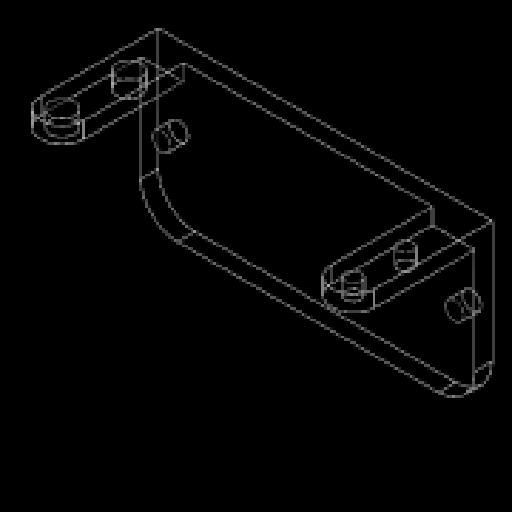
# Autodesk Inventor part: M3RCServoMountBracket
Saved by Autodesk Inventor 2025.2 (Build 292293000, 293)
## iProperties
Created: 2025-12-06
Part Number: M3RCServoMountBracket
Material: Generic
Document SubType Name: Modeling
Designer: valer
Density: 1 g/cm^3
Appearance: Default
Author: valer
Comments: https://www.amazon.com/dp/B0F372CLN4?ref=ppx_yo2ov_dt_b_fed_asin_title
Autodesk Inventor part; units mm, degrees
ref_plane "YZ Plane" through (0, 0, 0) normal (1, 0, 0) x (0, 1, 0)
ref_plane "XZ Plane" through (0, 0, 0) normal (0, 1, 0) x (-1, 0, 0)
ref_plane "XY Plane" through (0, 0, 0) normal (0, 0, 1) x (1, 0, 0)
sketch "Base" plane through (0, 0, 0) normal (0, 0, 1) x (1, 0, 0)
  line L0 (27.5, -13) -> (-27.5, -13)
  line L1 (-27.5, -13) -> (-27.5, 13)
  line L2 (-27.5, 13) -> (27.5, 13)
  line L3 (27.5, 13) -> (27.5, -13)
  line L4 (27.5, -13) -> (-27.5, 13) construction
  line L5 (-27.5, -13) -> (27.5, 13) construction
  line L6 (-27.5, 0) -> (27.5, 0) construction
  circle A0 centre (-24.15, 0) radius 1.5
  line L7 (0, -18.2) -> (0, 18.2) construction
  line L8 (-25.65, -1.5) -> (-22.65, -1.5) construction
  line L9 (-22.65, -1.5) -> (-22.65, 1.5)
  line L10 (-22.65, 1.5) -> (-25.65, 1.5) construction
  line L11 (-25.65, 1.5) -> (-25.65, -1.5) construction
  line L12 (-25.65, -1.5) -> (-22.65, 1.5) construction
  line L13 (-22.65, -1.5) -> (-25.65, 1.5) construction
  circle A1 centre (24.15, 0) radius 1.5
  point P0 (0, 0)
  dimension "d0" = 55
  dimension "d1" = 26
  dimension "d4" = 3
  dimension "d5" = 1.85
  constraints: 26 end point, 6 midpoint, 4 parallel, 2 centre point, 2 perpendicular, 2 tangent, 1 horizontal, 1 point on line, 1 symmetric about line, 1 other
  measures "d0" distance of L0.start L0.end
  measures "d1" distance of L0.end L1.end
  measures "d4" diameter of A0
  measures "d5" distance between parallel lines of L1 L11
extrude "BaseFeature" add sketch "Base" along normal blind 2.88
fillet "BaseFilletsFeature" radius 6 2 edges at (-27.5, -13, 1.44) (27.5, -13, 1.44)
sketch "ServoMount" plane through (0, 0, 2.88) normal (0, 0, 1) x (1, 0, 0)
  line L0 (27.5, 13) -> (-27.5, 13) projected
  line L1 (-27.5, 13) -> (-27.5, -7) projected
  line L2 (27.5, -7) -> (27.5, 13) projected
  line L3 (-27.5, 13) -> (-20.5, 13)
  line L4 (-20.5, 13) -> (-20.5, 10.35)
  line L5 (-20.5, 10.35) -> (-27.5, 10.35)
  line L6 (-27.5, 10.35) -> (-27.5, 13)
  line L7 (0, -18.2) -> (0, 18.2) construction
  line L8 (20.5, 13) -> (20.5, 10.35)
  line L9 (20.5, 10.35) -> (27.5, 10.35)
  point P0 (0, 0)
  point P1 (-24, 13)
  dimension "d7" = 2.65
  dimension "d8" = 7
  constraints: 12 end point, 3 symmetric about line, 2 parallel, 1 horizontal, 1 midpoint, 1 perpendicular
  measures "d7" distance from line of point (-24, 13) L5
  measures "d8" distance of L4.end L5.end
extrude "ServoMountFEature" add sketch "ServoMount" along normal blind 20
sketch "ServoMountProfile" plane through (-27.5, 10.35, 2.88) normal (0, -1, 0) x (1, 0, 0)
  line L0 (7, 0) -> (0, 0) projected
  line L1 (7, 0) -> (7, 20) projected
  line L2 (0, 20) -> (7, 20) projected
  line L3 (0, 0) -> (0, 20) projected
  line L4 (27.5, -7.456) -> (27.5, 24.576) construction
  circle A0 centre (3.5, 16.5) radius 3.5
  line L5 (3.5, 20) -> (3.5, 0) construction
  line L6 (0, 20) -> (7, 20) projected
  line L7 (0, 0) -> (0, 20) projected
  circle A1 centre (51.5, 16.5) radius 3.5
  line L8 (48, 0) -> (48, 20) projected
  line L9 (48, 20) -> (55, 20) projected
  line L10 (55, 0) -> (55, 20) projected
  point P0 (27.5, -2.88)
  point P1 (55, 16.5)
  point P2 (51.5, 20)
  point P3 (48, 16.5)
  point P4 (0, 16.5)
  point P5 (3.5, 20)
  point P6 (7, 16.5)
  constraints: 2 centre point, 2 end point, 2 midpoint, 2 tangent, 1 point on line, 1 symmetric about line, 1 other
extrude "ServoMountProfileFeature" cut sketch "ServoMountProfile" against normal blind 20 contours A0 L2 L1 | L3 L2 A0 | A1 L9 L10 | A1 L8 L9
sketch "ServoMountHoles" plane through (-27.5, 10.35, 2.88) normal (0, -1, 0) x (1, 0, 0)
  arc A0 (7, 16.5) -> (0, 16.5) centre (3.5, 16.5) ccw construction
  line L0 (0, 0) -> (0, 16.5) construction
  line L1 (7, 0) -> (0, 0) construction
  line L2 (7, 0) -> (7, 16.5) construction
  line L3 (27.5, 24.576) -> (27.5, -7.456) construction
  circle A1 centre (51.5, 16.5) radius 1.25
  circle A2 centre (51.5, 7.89) radius 1.25
  arc A3 (2.1771, 4) -> (2.1771, 7) centre (3.5, 5.5) ccw construction
  arc A4 (2.1771, 15) -> (2.1771, 18) centre (3.5, 16.5) ccw construction
  circle A5 centre (3.5, 5.5) radius 2
  arc A6 (7, 16.5) -> (0, 16.5) centre (3.5, 16.5) ccw projected
  circle A7 centre (3.5, 16.5) radius 2
  point P0 (27.5, -2.88)
  dimension "d17" = 4
  dimension "d18" = 4
  constraints: 4 centre point, 2 coincident
  measures "d17" diameter of A5
  measures "d18" diameter of A7
extrude "ServoMountHolesFeature" cut sketch "ServoMountHoles" against normal through all
body "Solid1"
